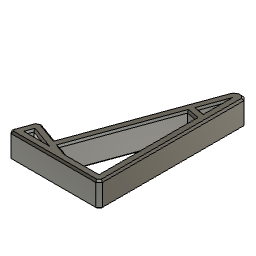
3D Printable Stand v1.0 (Autodesk Fusion 360 design; units mm, degrees)
Autodesk Fusion 360 part; units mm, degrees
sketch "Sketch1" plane through (0, 0, 0) normal (0, 0, 1) x (1, 0, 0)
  line L0 (0, 0) -> (5.1303, 14.0954)
  line L1 (0, 0) -> (15, 0) construction
  line L2 (5.1303, 14.0954) -> (19.2257, 8.9651)
  line L3 (5.1303, 14.0954) -> (20.1303, 14.0954) construction
  line L4 (19.2257, 8.9651) -> (46.5873, 84.1405)
  line L5 (19.2257, 8.9651) -> (99.2257, 8.9651) construction
  line L6 (46.5873, 84.1405) -> (55, 84.1405)
  line L7 (55, 84.1405) -> (55, 0)
  line L8 (55, 0) -> (0, 0)
  dimension "d1" = 70
  dimension "d2" = 15
  dimension "d3" = 20
  dimension "d4" = 15
  dimension "d5" = 70
  dimension "d6" = 80
  constraint horizontal L1
  constraint coincident L0.start L1.start
  constraint horizontal L3
  constraint horizontal L5
  constraint horizontal L6
  constraint perpendicular L6 L7
  constraint perpendicular L7 L8
  measures "d1" angle of L0 L1
  measures "d2" distance of L0.start L0.end
  measures "d3" angle of L2 L3
  measures "d4" distance of L0.end L2.end
  measures "d5" angle of L4 L5
  measures "d6" distance of L2.end L4.end
extrude "Extrude1" add sketch "Sketch1" along normal blind 15
sketch "Sketch2" plane through (0, 0, 15) normal (0, 0, 1) x (-1, 0, 0)
  line L0 (-55, 0) -> (-55, -84.1405)
  line L1 (-55, -84.1405) -> (-46.5873, -84.1405)
  line L2 (-46.5873, -84.1405) -> (-19.2257, -8.9651)
  line L3 (-19.2257, -8.9651) -> (-5.1303, -14.0954)
  line L4 (-5.1303, -14.0954) -> (0, 0)
  line L5 (0, 0) -> (-55, 0)
  line L6 (-23.9242, -7.255) -> (-49.9527, -78.7679)
  line L7 (-23.9242, -7.255) -> (52.1783, -7.255) construction
  line L8 (-49.9527, -78.7679) -> (-49.9527, -5)
  line L9 (-23.9242, -7.255) -> (-30.1197, -5)
  line L10 (-23.9242, -7.255) -> (-17.331, -7.255) construction
  line L11 (-49.9527, -5) -> (-30.1197, -5)
  dimension "d13" = 5
  dimension "d14" = 110
  dimension "d15" = 160
  constraint horizontal L7
  constraint perpendicular L5 L8
  constraint horizontal L10
  constraint perpendicular L8 L11
  measures "d13" distance of L2.end L6.start
  measures "d14" angle of L6 L7
  measures "d15" angle of L9 L10
extrude "Extrude2" cut sketch "Sketch2" against normal blind 78 contours L6 L8 L9 L11
sketch "Sketch3" plane through (0, 0, 15) normal (0, 0, 1) x (-1, 0, 0)
  line L0 (-49.9527, -5) -> (-30.1197, -5)
  line L1 (-30.1197, -5) -> (-23.9242, -7.255)
  line L2 (-23.9242, -7.255) -> (-49.9527, -78.7679)
  line L3 (-49.9527, -78.7679) -> (-49.9527, -5)
  line L4 (-55, 0) -> (-55, -84.1405)
  line L5 (-55, -84.1405) -> (-46.5873, -84.1405)
  line L6 (-46.5873, -84.1405) -> (-19.2257, -8.9651)
  line L7 (-19.2257, -8.9651) -> (-5.1303, -14.0954)
  line L8 (-5.1303, -14.0954) -> (0, 0)
  line L9 (0, 0) -> (-55, 0)
  line L10 (-7.1358, -4.9864) -> (-15.5382, -4.9864)
  line L11 (-7.1358, -4.9864) -> (-8.1187, -7.6868)
  line L12 (-8.1187, -7.6868) -> (-15.5382, -4.9864)
  constraint perpendicular L11 L12
extrude "Extrude3" cut sketch "Sketch3" against normal blind 57 contours L10 L11 L12
chamfer "Chamfer1" distance 2 angle 45 1 edges at (0, 0, 7.5)
chamfer "Chamfer2" distance 2 angle 45 1 edges at (55, 0, 7.5)
chamfer "Chamfer3" distance 2 angle 45 1 edges at (5.1303, 14.0954, 7.5)
chamfer "Chamfer8" distance 16 angle 45 1 edges at (49.9527, 78.7679, 7.5)
sketch "Sketch4" plane through (0, 0, 15) normal (0, 0, 1) x (-1, 0, 0)
  line L0 (-49.9527, -5) -> (-30.1197, -5)
  line L1 (-30.1197, -5) -> (-23.9242, -7.255)
  line L2 (-23.9242, -7.255) -> (-44.4804, -63.7328)
  line L3 (-44.4804, -63.7328) -> (-49.9527, -62.7679)
  line L4 (-49.9527, -62.7679) -> (-49.9527, -5)
  line L5 (-8.1187, -7.6868) -> (-15.5382, -4.9864)
  line L6 (-15.5382, -4.9864) -> (-7.1358, -4.9864)
  line L7 (-7.1358, -4.9864) -> (-8.1187, -7.6868)
  line L8 (-49.9527, -78.7679) -> (-46.2169, -68.5038)
  line L9 (-49.9527, -78.7679) -> (-49.9527, -67.8451)
  line L10 (-46.2169, -68.5038) -> (-49.9527, -67.8451)
  line L11 (-7.0097, -13.4113) -> (-4.4463, -12.216)
  line L12 (-4.4463, -12.216) -> (-0.684, -1.8794)
  line L13 (-0.684, -1.8794) -> (-2, 0)
  line L14 (-2, 0) -> (-53, 0)
  line L15 (-53, 0) -> (-55, -2)
  line L16 (-55, -2) -> (-55, -84.1405)
  line L17 (-55, -84.1405) -> (-46.5873, -84.1405)
  line L18 (-46.5873, -84.1405) -> (-19.2257, -8.9651)
  line L19 (-19.2257, -8.9651) -> (-7.0097, -13.4113)
extrude "Extrude4" cut sketch "Sketch4" against normal blind 36 contours L8 L9 L10
chamfer "Chamfer9" distance 1 angle 45 5 edges at (34.2023, 35.4939, 15) (27.0219, 6.1275, 15) (40.0362, 5, 15) (49.9527, 33.884, 15) (47.2166, 63.2504, 15)
chamfer "Chamfer10" distance 1 angle 45 5 edges at (49.9527, 33.884, 0) (47.2166, 63.2504, 0) (34.2023, 35.4939, 0) (27.0219, 6.1275, 0) (40.0362, 5, 0)
chamfer "Chamfer11" distance 1 angle 45 3 edges at (11.337, 4.9864, 15) (11.8284, 6.3366, 15) (7.6272, 6.3366, 15)
extrude "Extrude5" add 1 faces at (49.3915, 84.1405, 5) along direction (0, 1, 0) blind 5
sketch "Sketch5" plane through (0, 0, 15) normal (0, 0, 1) x (-1, 0, 0)
  line L0 (-50.9527, -63.607) -> (-50.9527, -4)
  line L1 (-50.9527, -4) -> (-29.9434, -4)
  line L2 (-29.9434, -4) -> (-22.6424, -6.6573)
  line L3 (-22.6424, -6.6573) -> (-43.8277, -64.8634)
  line L4 (-43.8277, -64.8634) -> (-50.9527, -63.607)
  line L5 (-49.9527, -67.8451) -> (-46.2169, -68.5038)
  line L6 (-46.2169, -68.5038) -> (-49.9527, -78.7679)
  line L7 (-49.9527, -78.7679) -> (-49.9527, -67.8451)
  line L8 (-7.0097, -13.4113) -> (-4.4463, -12.216)
  line L9 (-4.4463, -12.216) -> (-0.684, -1.8794)
  line L10 (-0.684, -1.8794) -> (-2, 0)
  line L11 (-2, 0) -> (-53, 0)
  line L12 (-53, 0) -> (-55, -2)
  line L13 (-55, -2) -> (-55, -89.1405)
  line L14 (-55, -89.1405) -> (-46.5873, -89.1405)
  line L15 (-46.5873, -89.1405) -> (-46.5873, -84.1405)
  line L16 (-46.5873, -84.1405) -> (-19.2257, -8.9651)
  line L17 (-19.2257, -8.9651) -> (-7.0097, -13.4113)
  line L18 (-5.7076, -3.9864) -> (-7.521, -8.9685)
  line L19 (-7.521, -8.9685) -> (-21.2094, -3.9864)
  line L20 (-21.2094, -3.9864) -> (-5.7076, -3.9864)
  line L21 (-46.5873, -84.1405) -> (-48.4072, -89.1405)
  line L22 (-46.5873, -84.1405) -> (-41.2664, -84.1405) construction
  dimension "d43" = 110
  constraint horizontal L22
  constraint coincident L15.end L16.start
  constraint coincident L14 L21.end
  measures "d43" angle of L21 L22
extrude "Extrude6" cut sketch "Sketch5" against normal blind 20 contours L14 L15 L21
chamfer "Chamfer12" distance 1 angle 45 3 edges at (48.0848, 73.6359, 15) (49.9527, 73.3065, 15) (48.0848, 68.1744, 15)
chamfer "Chamfer13" distance 2 angle 45 2 edges at (48.4072, 89.1405, 7.5) (55, 89.1405, 7.5)
chamfer "Chamfer14" distance 1 angle 45 11 edges at (5.728, 12.8137, 15) (2.5652, 7.0477, 15) (1.342, 0.9397, 15) (27.5, 0, 15) (13.1177, 11.1882, 15) (33.4744, 48.1131, 15) (55, 44.5702, 15) (54, 1, 15) (54, 88.1405, 15) (51.7036, 89.1405, 15) (49.0651, 88.2008, 15)
chamfer "Chamfer15" distance 1 angle 45 11 edges at (55, 44.5702, 0) (54, 88.1405, 0) (51.7036, 89.1405, 0) (49.0651, 88.2008, 0) (33.4744, 48.1131, 0) (13.1177, 11.1882, 0) (5.728, 12.8137, 0) (2.5652, 7.0477, 0) (1.342, 0.9397, 0) (27.5, 0, 0) (54, 1, 0)
chamfer "Chamfer16" distance 1 angle 45 3 edges at (49.9527, 73.3065, 0) (48.0848, 73.6359, 0) (48.0848, 68.1744, 0)
chamfer "Chamfer17" distance 1 angle 45 3 edges at (11.337, 4.9864, 0) (11.8284, 6.3366, 0) (7.6272, 6.3366, 0)
